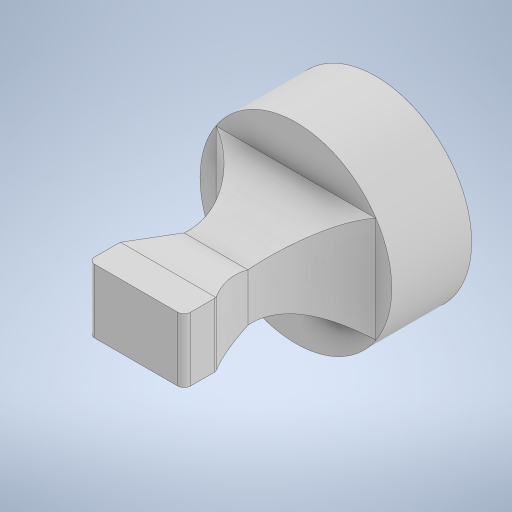
# Autodesk Inventor part: Arm 6 v0.1
Saved by Autodesk Inventor 2023 (Build 270158000, 158)
## iProperties
Created: 2024-06-24
Part Number: Arm 6 v0.1
Material: Generic
Document SubType Name: Modeling
Designer: Swoby
Density: 1 g/cm^3
Appearance: Default
Author: Swoby
Autodesk Inventor part; units mm, degrees
ref_plane "YZ Plane" through (0, 0, 0) normal (1, 0, 0) x (0, 1, 0)
ref_plane "XZ Plane" through (0, 0, 0) normal (0, 1, 0) x (-1, 0, 0)
ref_plane "XY Plane" through (0, 0, 0) normal (0, 0, 1) x (1, 0, 0)
sketch "Sketch1" plane through (0, 0, 0) normal (0, 0, 1) x (1, 0, 0)
  circle A0 centre (0, 0) radius 25
  circle A1 centre (0, 0) radius 30
  dimension "d0" = 50
  dimension "d1" = 60
  constraints: 3 coincident, 2 centre point
  measures "d0" diameter of A0
  measures "d1" diameter of A1
extrude "Extrusion1" add sketch "Sketch1" along normal blind 20
sketch "Sketch2" plane through (0, 0, 20) normal (0, 0, 1) x (1, 0, 0)
  circle A0 centre (0, 0) radius 30 projected
extrude "Extrusion2" add sketch "Sketch2" along normal blind 5
sketch "Sketch3" plane through (0, 0, 0) normal (0, 1, 0) x (-1, 0, 0)
  line L0 (30, 25) -> (-30, 25) projected
  arc A0 (-25, 25) -> (-10, 50) centre (-34.9158, 47.9495) ccw
  arc A1 (10, 50) -> (25, 25) centre (34.9158, 47.9495) ccw
  line L1 (-25, 20) -> (-25, 0) projected
  line L2 (25, 20) -> (25, 0) projected
  line L3 (-10, 50) -> (10, 50)
  arc A2 (-10, 50) -> (-23.3636, 64.782) centre (-26.3452, 48.6548) ccw construction
  line L4 (-10, 50) -> (-25, 65) construction
  line L5 (-10, 50) -> (11.2132, 50) construction
  arc A3 (23.3636, 64.782) -> (10, 50) centre (26.3452, 48.6548) ccw construction
  line L6 (-23, 75) -> (13, 75) construction
  line L7 (-25, 66.7486) -> (-25, 73) construction
  line L8 (25, 66.7486) -> (25, 73) construction
  arc A4 (-23, 75) -> (-25, 73) centre (-23, 73) ccw construction
  arc A5 (-25, 66.7486) -> (-23.3636, 64.782) centre (-23, 66.7486) ccw construction
  arc A6 (23.3636, 64.782) -> (25, 66.7486) centre (23, 66.7486) ccw construction
  arc A7 (25, 73) -> (23, 75) centre (23, 73) ccw construction
  line L9 (-13, 75) -> (15, 75)
  line L10 (15, 73) -> (15, 65.5675)
  line L11 (15, 65) -> (-15, 65) construction
  line L12 (-15, 65.5675) -> (-15, 73)
  arc A8 (-10, 50) -> (-14.7104, 64.531) centre (-43.196, 47.268) ccw
  arc A9 (14.7104, 64.531) -> (10, 50) centre (43.196, 47.268) ccw
  arc A10 (-15, 65.5675) -> (-14.7104, 64.531) centre (-13, 65.5675) ccw
  arc A11 (-13, 75) -> (-15, 73) centre (-13, 73) ccw
  arc A12 (15, 73) -> (13, 75) centre (13, 73) ccw
  arc A13 (14.7104, 64.531) -> (15, 65.5675) centre (13, 65.5675) ccw
  point P0 (0, 0)
  point P1 (25, 65)
  point P2 (-15, 75)
  dimension "d6" = 25
  dimension "d7" = 25
  dimension "d8" = 20
  dimension "d9" = 10
  dimension "d10" = 25
  dimension "d11" = 135
  dimension "d12" = 135
  dimension "d13" = 10
  dimension "d14" = 2
  dimension "d33" = 50
  dimension "d34" = 30
  dimension "d35" = 15
  dimension "d36" = 10
  dimension "d37" = 15
  dimension "d38" = 2
  constraints: 32 point on circle, 20 end point, 14 centre point, 14 point on line, 10 tangent, 3 equal radius, 3 horizontal, 2 parallel, 1 perpendicular
  measures "d6" distance between parallel lines of L0 L3
  measures "d7" radius of A1
  measures "d8" distance of L3.start L3.end
  measures "d9" horizontal distance of point (0, 0) L3.end
  measures "d10" radius of A0
  measures "d11" angle of L5 L4
  measures "d13" distance from line of L4.end L6
  measures "d14" radius of A4
  measures "d33" distance between parallel lines of L8 L7
  measures "d34" distance of point (-15, 75) L9.end
  measures "d35" distance from line of point (0, 0) L12
  measures "d36" distance of L9.end L11.start
  measures "d37" distance between parallel lines of L3 L11
  measures "d38" radius of A10
extrude "Extrusion3" add sketch "Sketch3" along normal mid plane 33
sketch "Sketch6" plane through (0, 0, 0) normal (1, 0, 0) x (0, 1, 0)
  line L0 (16.5, 25) -> (-16.5, 25) projected
  line L1 (16.5, 50) -> (-16.5, 50) projected
  line L2 (0, 50) -> (7.5, 50)
  line L3 (0, 50) -> (-7.5, 50)
  line L4 (-16.5, 25) -> (-16.5, 50) projected
  arc A0 (-16.5, 25) -> (-7.5, 50) centre (-47.499, 50.2796) ccw
  line L5 (16.5, 50) -> (16.5, 25) projected
  arc A1 (7.5, 50) -> (16.5, 25) centre (47.499, 50.2796) ccw
  line L6 (-16.5, 75) -> (16.5, 75) projected
  line L7 (10, 75) -> (-10, 75)
  line L8 (-10, 75) -> (-10, 65)
  line L9 (-10, 65) -> (10, 65)
  line L10 (10, 65) -> (10, 75)
  arc A2 (7.5, 50) -> (10, 65) centre (-36.25, 65) ccw
  arc A3 (-10, 65) -> (-7.5, 50) centre (36.25, 65) ccw
  line L11 (16.5, 64.531) -> (16.5, 50) projected
  line L12 (16.5, 50) -> (16.5, 75)
  line L13 (-16.5, 50) -> (-16.5, 64.531) projected
  line L14 (-16.5, 75) -> (-16.5, 50)
  point P0 (0, 0)
  dimension "d39" = 7.5
  dimension "d40" = 7.5
  dimension "d41" = 40
  dimension "d42" = 40
  dimension "d43" = 20
  dimension "d44" = 10
  dimension "d46" = 20
  dimension "d47" = 10
  dimension "d48" = 10
  constraints: 16 end point, 8 point on circle, 4 centre point, 4 point on line, 2 collinear, 2 tangent, 1 midpoint, 1 perpendicular
  measures "d39" distance of L2.start L2.end
  measures "d40" distance of L2.start L3.end
  measures "d41" radius of A1
  measures "d42" radius of A0
  measures "d43" distance of L7.start L7.end
  measures "d44" distance of L7.end L8.end
  measures "d46" distance of L8.end L9.end
  measures "d47" distance of L9.end L7.start
  measures "d48" distance from line of L10 point (0, 0)
extrude "Extrusion6" cut sketch "Sketch6" along normal through all both and the other way through all contours A1 L1 L5 | L4 L1 A0 | L1 A2 L10 L6 L12 L11 | L13 L14 L6 L8 A3 L1
body "Solid1"
